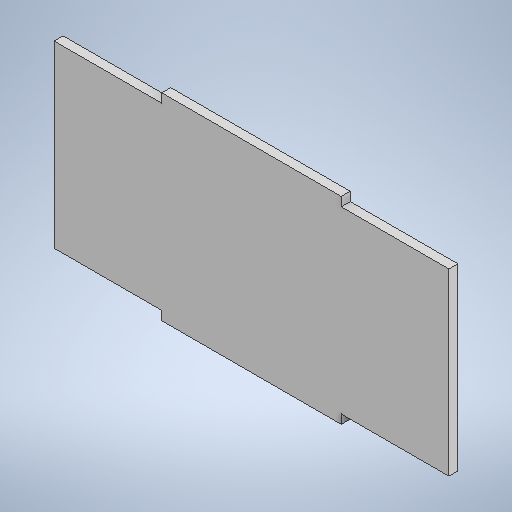
# Autodesk Inventor part: front
Saved by Autodesk Inventor 2025.3 (Build 293356030, 356C)
## iProperties
Created: 2026-06-26
Part Number: front
Material: Generic
Document SubType Name: Modeling
Designer: user
Density: 1 g/cm^3
Appearance: Default
Author: user
Autodesk Inventor part; units mm, degrees
ref_plane "YZ Plane" through (0, 0, 0) normal (1, 0, 0) x (0, 1, 0)
ref_plane "XZ Plane" through (0, 0, 0) normal (0, 1, 0) x (-1, 0, 0)
ref_plane "XY Plane" through (0, 0, 0) normal (0, 0, 1) x (1, 0, 0)
sketch "Sketch1" plane through (0, 0, 0) normal (0, 0, 1) x (1, 0, 0)
  line L0 (0, 0) -> (220, 0)
  line L1 (220, 0) -> (220, 100)
  line L2 (220, 100) -> (0, 100)
  line L3 (0, 100) -> (0, 0)
  line L4 (60, 0) -> (160, 0)
  line L5 (160, 0) -> (160, -5)
  line L6 (160, -5) -> (60, -5)
  line L7 (60, -5) -> (60, 0)
  line L8 (60, 100) -> (160, 100)
  line L9 (160, 100) -> (160, 105)
  line L10 (160, 105) -> (60, 105)
  line L11 (60, 105) -> (60, 100)
  point P0 (0, 20)
  point P1 (160, 0)
  point P2 (60, 102.5)
  dimension "d0" = 220
  dimension "d1" = 100
  dimension "d2" = 100
  dimension "d3" = 5
  dimension "d8" = 60
  dimension "d9" = 5
  dimension "d10" = 100
  dimension "d11" = 60
  constraints: 24 end point, 6 parallel, 3 horizontal, 3 perpendicular, 3 point on line, 1 midpoint
  measures "d0" distance of L2.end L1.end
  measures "d1" distance of L1.end L0.end
  measures "d2" distance of L5.end L6.end
  measures "d3" distance of L4.end L5.end
  measures "d8" distance from line of L7 L0.start
  measures "d9" distance of L9.end L8.end
  measures "d10" distance between parallel lines of L9 L11
  measures "d11" distance from line of point (60, 102.5) L3
extrude "Extrusion1" add sketch "Sketch1" along normal blind 5
body "Solid1"
